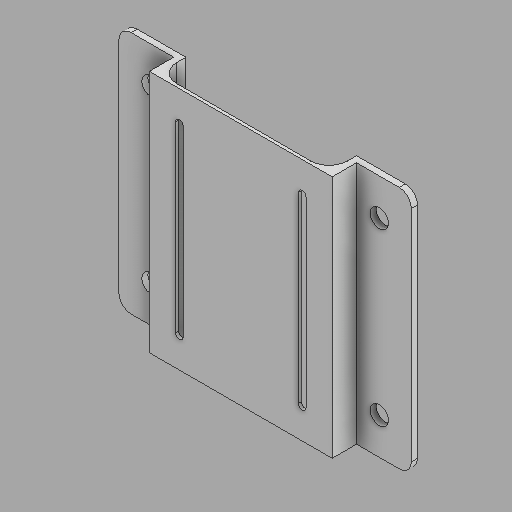
# Autodesk Inventor part: RC_CAR_LIDAR_PLATE
Saved by Autodesk Inventor 2025.2 (Build 292293000, 293)
## iProperties
Created: 2026-01-02
Part Number: RC_CAR_LIDAR_PLATE
Material: Generic
Document SubType Name: Modeling
Designer: Ben
Density: 1 g/cm^3
Appearance: Default
Author: Ben
Autodesk Inventor part; units mm, degrees
ref_plane "YZ Plane" through (0, 0, 0) normal (1, 0, 0) x (0, 1, 0)
ref_plane "XZ Plane" through (0, 0, 0) normal (0, 1, 0) x (-1, 0, 0)
ref_plane "XY Plane" through (0, 0, 0) normal (0, 0, 1) x (1, 0, 0)
sketch "Sketch1" plane through (0, 0, 0) normal (0, 0, 1) x (1, 0, 0)
  line L0 (-38.1, -31.75) -> (38.1, -31.75)
  line L1 (38.1, -31.75) -> (38.1, 31.75)
  line L2 (38.1, 31.75) -> (-38.1, 31.75)
  line L3 (-38.1, 31.75) -> (-38.1, -31.75)
  line L4 (-38.1, -31.75) -> (38.1, 31.75) construction
  line L5 (38.1, -31.75) -> (-38.1, 31.75) construction
  point P0 (0, 0)
  dimension "d0" = 76.2
  dimension "d1" = 63.5
  constraints: 12 end point, 2 midpoint, 2 parallel, 1 horizontal, 1 perpendicular
  measures "d0" distance of L1.end L2.end
  measures "d1" distance of L2.end L0.start
extrude "Extrusion1" add sketch "Sketch1" along normal blind 1.5875
sketch "Sketch2" plane through (0, 0, 1.5875) normal (0, 0, 1) x (1, 0, 0)
  line L0 (0, -44.45) -> (0, 44.45) projected
  line L1 (-53.34, 0) -> (53.34, 0) projected
  line L2 (38.1, 31.75) -> (-38.1, 31.75) projected
  point P0 (0, 0)
  point P1 (-29.765, 22.225)
  point P2 (29.765, 22.225)
  point P3 (29.765, -22.225)
  point P4 (-29.765, -22.225)
  dimension "d4" = 59.53
  dimension "d5" = 9.525
  constraints: 3 symmetric about line
  measures "d4" distance of point (29.765, 22.225) point (-29.765, 22.225)
  measures "d5" distance from line of L2 point (-29.765, 22.225)
hole "Hole1" at (-29.765, -22.225, 1.5875) at (-29.765, 22.225, 1.5875) at (29.765, 22.225, 1.5875) at (29.765, -22.225, 1.5875) direction (0, 0, -1) diameter 4.7752 end through all
sketch "Sketch4" plane through (0, 0, 1.5875) normal (0, 0, 1) x (1, 0, 0)
  line L0 (38.1, 31.75) -> (-38.1, 31.75) projected
  line L1 (-23.8125, -31.75) -> (23.8125, -31.75)
  line L2 (23.8125, -31.75) -> (23.8125, 31.75)
  line L3 (23.8125, 31.75) -> (-23.8125, 31.75)
  line L4 (-23.8125, 31.75) -> (-23.8125, -31.75)
  line L5 (-23.8125, -31.75) -> (23.8125, 31.75) construction
  line L6 (23.8125, -31.75) -> (-23.8125, 31.75) construction
  point P0 (0, 0)
  point P1 (-23.8125, 31.75)
  dimension "d13" = 47.625
  constraints: 12 end point, 2 midpoint, 2 parallel, 1 horizontal, 1 perpendicular, 1 point on line
  measures "d13" distance of L1.start L1.end
extrude "Extrusion2" add sketch "Sketch4" along normal blind 6.35
sketch "Sketch5" plane through (-38.1, -31.75, 0) normal (0, -1, 0) x (1, 0, 0)
  line L0 (76.2, 0) -> (0, 0) projected
  line L1 (15.875, 7.1437) -> (60.325, 7.1437)
  line L2 (60.325, 7.1437) -> (60.325, 0)
  line L3 (60.325, 0) -> (15.875, 0)
  line L4 (15.875, 0) -> (15.875, 7.1437)
  line L5 (14.2875, 7.9375) -> (61.9125, 7.9375) projected
  line L6 (14.2875, 1.5875) -> (14.2875, 7.9375) projected
  line L7 (61.9125, 1.5875) -> (61.9125, 7.9375) projected
  point P0 (38.1, 0)
  dimension "d16" = 0.7937
  dimension "d17" = 1.5875
  dimension "d18" = 1.5875
  constraints: 8 end point, 2 parallel, 1 horizontal, 1 perpendicular, 1 point on line
  measures "d16" distance between parallel lines of L5 L1
  measures "d17" distance between parallel lines of L6 L4
  measures "d18" distance between parallel lines of L7 L2
extrude "Extrusion3" cut sketch "Sketch5" along normal through all both and the other way through all
sketch "Sketch6" plane through (0, 0, 7.9375) normal (0, 0, 1) x (1, 0, 0)
  line L0 (-16, -23.8125) -> (-16, 23.8125) construction
  line L1 (-15, -23.8125) -> (-15, 23.8125)
  line L2 (-17, 23.8125) -> (-17, -23.8125)
  arc A0 (-17, -23.8125) -> (-15, -23.8125) centre (-16, -23.8125) ccw
  arc A1 (-15, 23.8125) -> (-17, 23.8125) centre (-16, 23.8125) ccw
  line L3 (16, -23.8125) -> (16, 23.8125) construction
  line L4 (15, -23.8125) -> (15, 23.8125)
  line L5 (17, 23.8125) -> (17, -23.8125)
  arc A2 (15, -23.8125) -> (17, -23.8125) centre (16, -23.8125) ccw
  arc A3 (17, 23.8125) -> (15, 23.8125) centre (16, 23.8125) ccw
  line L6 (0, -44.45) -> (0, 44.45) projected
  line L7 (-53.34, 0) -> (53.34, 0) projected
  line L8 (23.8125, 31.75) -> (-23.8125, 31.75) projected
  point P0 (0, 0)
  point P1 (-16, 0)
  point P2 (16, 0)
  dimension "d21" = 32
  dimension "d22" = 2
  dimension "d23" = 7.9375
  constraints: 16 end point, 8 point on circle, 8 tangent, 4 centre point, 3 parallel, 2 horizontal alignment, 2 midpoint, 1 equal radius, 1 symmetric about line, 1 vertical, 1 other
  measures "d21" distance between parallel lines of L3 L0
  measures "d22" distance between parallel lines of L2 L1
  measures "d23" distance from line of L8 L0.end
extrude "Extrusion4" cut sketch "Sketch6" against normal through all
fillet "Fillet1" radius 3.175 4 edges at (-38.1, 31.75, 0.7937) (-38.1, -31.75, 0.7937) (38.1, -31.75, 0.7937) (38.1, 31.75, 0.7937)
fillet "Fillet2" radius 4.7625 2 edges at (-22.225, 0, 7.1437) (22.225, 0, 7.1437)
body "Solid1"
